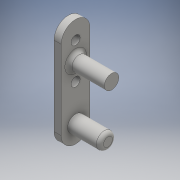
# Autodesk Inventor part: cube_Holder
Saved by Autodesk Inventor 2016 (Build 200138000, 138)
## iProperties
Created: 2024-07-21
Part Number: cube_Holder
Material: Generic
Document SubType Name: Modeling
Designer: Dell
Density: 1 g/cm^3
Appearance: Default
Author: Dell
Autodesk Inventor part; units mm, degrees
ref_plane "YZ Plane" through (0, 0, 0) normal (1, 0, 0) x (0, 1, 0)
ref_plane "XZ Plane" through (0, 0, 0) normal (0, 1, 0) x (-1, 0, 0)
ref_plane "XY Plane" through (0, 0, 0) normal (0, 0, 1) x (1, 0, 0)
sketch "Sketch1" plane through (0, 0, 0) normal (1, 0, 0) x (0, 1, 0)
  line L0 (6.2348, 11.9337) -> (6.2348, 11.9337)
  line L1 (2.2348, 7.9337) -> (2.2348, -14.0663)
  line L2 (6.2348, -18.0663) -> (6.2348, -18.0663)
  line L3 (10.2348, -14.0663) -> (10.2348, 7.9337)
  circle A0 centre (6.2348, 6.9337) radius 1.25
  circle A1 centre (6.2348, -3.0663) radius 1.25
  circle A2 centre (6.2348, -13.0663) radius 2.25
  arc A3 (6.2348, -18.0663) -> (10.2348, -14.0663) centre (6.2348, -14.0663) ccw
  arc A4 (2.2348, -14.0663) -> (6.2348, -18.0663) centre (6.2348, -14.0663) ccw
  arc A5 (6.2348, 11.9337) -> (2.2348, 7.9337) centre (6.2348, 7.9337) ccw
  arc A6 (10.2348, 7.9337) -> (6.2348, 11.9337) centre (6.2348, 7.9337) ccw
  point P0 (0, 0)
  point P1 (10.2348, 11.9337)
  point P2 (2.2348, 11.9337)
  point P3 (10.2348, -18.0663)
  dimension "d0" = 30
  dimension "d1" = 8
  dimension "d2" = 10
  dimension "d3" = 20
  dimension "d4" = 5
  dimension "d5" = 4.5
  dimension "d6" = 2.5
  dimension "d7" = 2.5
  dimension "d8" = 4
  constraints: 8 end point, 8 point on circle, 8 tangent, 7 centre point, 6 point on line, 3 equal radius, 2 parallel, 1 horizontal, 1 perpendicular
  measures "d0" distance of point (10.235, -18.066) point (10.235, 11.934)
  measures "d1" distance of point (10.235, 11.934) point (2.235, 11.934)
  measures "d2" distance of A1.centre A0.centre
  measures "d3" distance of A0.centre A2.centre
  measures "d4" distance from line of L2 A2.centre
  measures "d5" diameter of A2
  measures "d6" diameter of A1
  measures "d7" diameter of A0
  measures "d8" radius of A3
extrude "Extrusion1" add sketch "Sketch1" along normal blind 2
sketch "Sketch2" plane through (2, 0, 0) normal (1, 0, 0) x (0, 0, -1)
  circle A0 centre (-1.9337, 6.2348) radius 2
  circle A1 centre (3.0663, 6.2348) radius 1.25 projected
  point P0 (0, 0)
  dimension "d11" = 4
  dimension "d12" = 5
  constraints: 1 centre point
  measures "d11" diameter of A0
  measures "d12" distance of A1.centre A0.centre
extrude "Extrusion2" add sketch "Sketch2" along normal blind 10 contours A0
fillet "Fillet1" radius 1 1 edges at (2, 6.2348, 3.9337)
sketch "Sketch4" plane through (2, 0, 0) normal (1, 0, 0) x (0, 0, -1)
  circle A0 centre (13.0663, 6.2348) radius 2.25 projected
  circle A1 centre (13.0663, 6.2348) radius 2.4
  point P0 (0, 0)
  dimension "d25" = 4.8
  constraints: 1 centre point, 1 coincident
  measures "d25" diameter of A1
extrude "Extrusion4" add sketch "Sketch4" along normal blind 9 and the other way blind 2 contours A0
fillet "Fillet2" radius 1 1 edges at (11, 6.2348, -10.8163)
body "Solid1"
